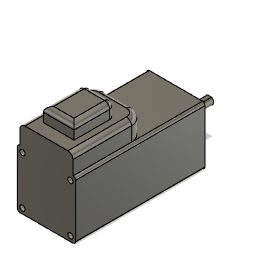
Mouting Plate BOB v17 (Autodesk Fusion 360 archive; units mm, degrees)
design "NEMA 23 Integrated Easy Servo Motor 130w"
Autodesk Fusion 360 part; units mm, degrees
sketch "Sketch1" plane through (0, 0, 0) normal (0, 0, 1) x (1, 0, 0)
  line L0 (0, 0) -> (57.15, 0)
  line L1 (57.15, 0) -> (57.15, 57.15)
  line L2 (57.15, 57.15) -> (0, 57.15)
  line L3 (0, 57.15) -> (0, 0)
  circle A0 centre (52.125, 52.125) radius 2.6
  line L4 (28.575, 0) -> (28.575, 57.15) construction
  line L5 (0, 28.575) -> (57.15, 28.575) construction
  circle A1 centre (5.025, 52.125) radius 2.6
  circle A2 centre (5.025, 5.025) radius 2.6
  circle A3 centre (52.125, 5.025) radius 2.6
  circle A4 centre (28.575, 28.575) radius 19.05
  line L6 (2.575, 57.15) -> (54.575, 57.15)
  line L7 (54.575, 57.15) -> (54.575, 76)
  line L8 (54.575, 76) -> (2.575, 76)
  line L9 (2.575, 76) -> (2.575, 57.15)
  circle A5 centre (28.575, 28.575) radius 4
  line L10 (26.6385, 32.075) -> (30.5115, 32.075)
  line L11 (13.575, 76) -> (43.575, 76)
  line L12 (43.575, 76) -> (43.575, 89.67)
  line L13 (43.575, 89.67) -> (13.575, 89.67)
  line L14 (13.575, 89.67) -> (13.575, 76)
  point P0 (47.5479, 45.3005)
  dimension "d1" = 57.15
  dimension "d2" = 57.15
  dimension "d3" = 5.2
  dimension "d5" = 5.2
  dimension "d6" = 47.1
  dimension "d8" = 5.2
  dimension "d10" = 47.1
  dimension "d12" = 5.2
  dimension "d13" = 47.1
  dimension "d14" = 47.1
  dimension "d15" = 38.1
  dimension "d16" = 76
  dimension "d17" = 8
  dimension "d19" = 3.5
  dimension "d20" = 52
  dimension "d21" = 13.67
  dimension "d22" = 30
  constraint horizontal L0
  constraint vertical L1
  constraint horizontal L2
  constraint vertical L3
  constraint coincident L0.start L3.end
  constraint midpoint L0 L4.start
  constraint midpoint L2 L4.end
  constraint midpoint L3 L5.start
  constraint midpoint L1 L5.end
  constraint symmetric A0 L4 A1
  constraint symmetric L5 A1.centre A2.centre
  constraint midpoint L5 A4.centre
  constraint horizontal L6
  constraint vertical L7
  constraint horizontal L8
  constraint vertical L9
  constraint coincident L2 L6.start
  constraint concentric A4 A5
  constraint coincident A5 L10.start
  constraint coincident A5 L10.end
  constraint perpendicular L4 L10
  constraint symmetric L4 L7 L9
  constraint horizontal L11
  constraint vertical L12
  constraint horizontal L13
  constraint vertical L14
  constraint coincident L8 L11.start
  constraint symmetric L4 L12 L14
  measures "d1" distance of L0.start L0.end
  measures "d2" distance of L0.start L2.end
  measures "d3" diameter of A0
  measures "d5" diameter of A1
  measures "d6" distance of A0.centre A1.centre
  measures "d8" diameter of A2
  measures "d10" distance of A1.centre A2.centre
  measures "d12" diameter of A3
  measures "d13" horizontal distance of A2.centre A3.centre
  measures "d14" distance of A0.centre A3.centre
  measures "d15" diameter of A4
  measures "d16" distance of L0 L8
  measures "d17" diameter of A5
  measures "d19" distance of L5 L10
  measures "d20" distance of L7.end L8.end
  measures "d21" distance of L11.start L13.end
  measures "d22" distance of L12.end L13.end
extrude "Extrude1" add sketch "Sketch1" along normal blind 127 contours L0 L1 L2 L3 L6 | A4 | A5 L10 | A5 L10
fillet "Fillet1" radius 2.5 4 edges at (57.15, 57.15, 63.5) (57.15, 0, 63.5) (0, 0, 63.5) (0, 57.15, 63.5)
extrude "Extrude2" add sketch "Sketch1" against normal blind 70 from surface at 127 contours L2 L6 L7 L8 L9 L11
fillet "Fillet2" radius 12.5 2 edges at (54.575, 66.575, 57) (2.575, 66.575, 57)
fillet "Fillet2" radius 5 3 edges at (54.575, 76, 92) (28.575, 76, 57) (2.575, 76, 92)
extrude "Extrude3" add sketch "Sketch1" along normal blind 40 from surface at 75 contours L8 L11 L12 L13 L14
fillet "Fillet3" radius 5 6 edges at (43.575, 89.67, 95) (43.575, 82.835, 75) (13.575, 82.835, 75) (28.575, 89.67, 75) (13.575, 89.67, 95) (28.575, 89.67, 115)
extrude "Extrude4" add sketch "Sketch1" against normal blind 2 contours A4 | A5 L10 | A5 L10
extrude "Extrude5" add sketch "Sketch1" against normal blind 33 contours A5 L10 picked at (29.5161, 29.5962)
extrude "Extrude6" add sketch "Sketch1" against normal blind 6 contours A5 L10 picked at (28.1041, 32.1557)
equation "d10 = d6"
equation "d12 = d3"
equation "d13 = d6"
equation "d14 = d6"
equation "d19 = 7.5 mm - ( d17 / 2 )"
equation "d44 = ( -1 * ( 33 - 27 ) ) * 1 mm"

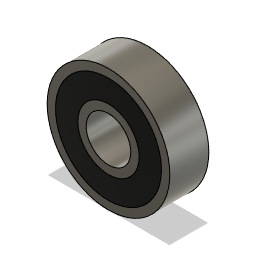
design "608 Bearings"
Autodesk Fusion 360 part; units mm, degrees
sketch "Sketch1" plane through (0, 0, 0) normal (0, 0, 1) x (1, 0, 0)
  circle A0 centre (0, 0) radius 11
  circle A1 centre (0, 0) radius 9.5
  circle A2 centre (0, 0) radius 4
  circle A3 centre (0, 0) radius 5.5
  dimension "d1" = 22
  dimension "d2" = -1.5
  dimension "d3" = 8
  dimension "d4" = 1.5
  constraint coincident A0.centre A1.centre
  measures "d1" diameter of A0
  measures "d3" diameter of A2
extrude "Extrude1" add sketch "Sketch1" along normal blind 7 makes body 1 at (5.4727, -0.5476, 4.6667) makes body 2 at (10.9453, -1.0952, 4.6667)
extrude "Extrude2" add sketch "Sketch1" along normal blind 7 separate body contours A1 makes body 3

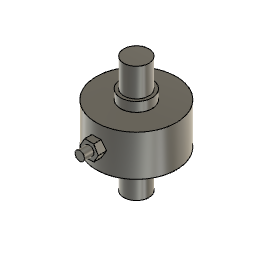
design "Load Cell Mini (200 kg)"
Autodesk Fusion 360 part; units mm, degrees
sketch "Boceto1" plane through (0, 0, 0) normal (0, 0, 1) x (1, 0, 0)
  circle A0 centre (0, 0) radius 12.7
  dimension "d1" = 25.4
  constraint coincident A0.centre origin
  measures "d1" diameter of A0
extrude "Extruir1" add sketch "Boceto1" along normal blind 13
sketch "Boceto2" plane through (0, 0, 13) normal (0, 0, 1) x (-1, 0, 0)
  circle A0 centre (0, 0) radius 12.7
  circle A1 centre (0, 0) radius 5
  dimension "d4" = 10
  constraint coincident A0.centre A1.centre
  measures "d4" diameter of A1
extrude "Extruir2" add sketch "Boceto2" along normal blind 3 contours A1
sketch "Boceto3" plane through (0, 0, 16) normal (0, 0, 1) x (-1, 0, 0)
  circle A0 centre (0, 0) radius 5
  circle A1 centre (0, 0) radius 4
  dimension "d7" = 8
  constraint coincident A0.centre A1.centre
  measures "d7" diameter of A1
extrude "Extruir3" add sketch "Boceto3" along normal blind 9 contours A1
sketch "Boceto4" plane through (0, 0, 0) normal (0, 0, -1) x (1, 0, 0)
  circle A0 centre (0, 0) radius 12.7
  circle A1 centre (0, 0) radius 4
  dimension "d10" = 8
  constraint coincident A0.centre A1.centre
  measures "d10" diameter of A1
extrude "Extruir4" add sketch "Boceto4" along normal blind 12 contours A1
sketch "Boceto5" plane through (0, 0, 0) normal (0, 1, 0) x (1, 0, 0)
  line L0 (-1.4434, -4) -> (-2.8868, -6.5)
  line L1 (-2.8868, -6.5) -> (-1.4434, -9)
  line L2 (-1.4434, -9) -> (1.4434, -9)
  line L3 (1.4434, -9) -> (2.8868, -6.5)
  line L4 (2.8868, -6.5) -> (1.4434, -4)
  line L5 (1.4434, -4) -> (-1.4434, -4)
  line L6 (-12.7, 0) -> (12.7, 0)
  point P0 (0, -6.5)
  dimension "d15" = 6.5
  dimension "d16" = 5
  measures "d15" distance of P0 L6
  measures "d16" distance of L2 L5
extrude "Extruir5" add sketch "Boceto5" against normal blind 15
sketch "Boceto6" plane through (0, -15, 0) normal (0, -1, 0) x (1, 0, 0)
  line L0 (-1.4434, 4) -> (1.4434, 4)
  line L1 (1.4434, 4) -> (2.8868, 6.5)
  line L2 (2.8868, 6.5) -> (1.4434, 9)
  line L3 (1.4434, 9) -> (-1.4434, 9)
  line L4 (-1.4434, 9) -> (-2.8868, 6.5)
  line L5 (-2.8868, 6.5) -> (-1.4434, 4)
  circle A0 centre (0, 6.5) radius 1.5
  dimension "d17" = 3
  measures "d17" diameter of A0
extrude "Extruir6" add sketch "Boceto6" along normal blind 3 contours A0

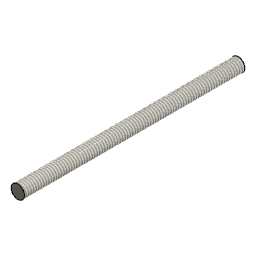
design "8mm T8 Lead Screw (130mm) v1"
Autodesk Fusion 360 part; units mm, degrees
sketch "Sketch1" plane through (0, 0, 0) normal (0, 0, 1) x (1, 0, 0)
  circle A0 centre (0, 0) radius 4
  dimension "d1" = 8
  constraint coincident A0.centre origin
  measures "d1" diameter of A0
extrude "Extrude1" add sketch "Sketch1" along normal blind 130
thread "Thread1" "ISO Metric Trapezoidal Threads 8.0 TR8x1.5 7e" major diameter 7.925 minor diameter 6.0605 pitch 1.5 angle 30 resizes the face on face at (3.9801, -0.3983, 43.3333)

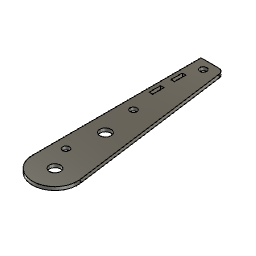
design "Pedal Inox"
Autodesk Fusion 360 part; units mm, degrees
sketch "Boceto1" plane through (0, 0, 0) normal (0, 0, 1) x (1, 0, 0)
  circle A0 centre (40.124, 0.0001) radius 5
  circle A1 centre (30, 20) radius 3
  line L0 (40.124, 0.0001) -> (40, -27.0971) construction
  line L1 (20.124, 0) -> (20.033, 149.9909)
  circle A2 centre (30, 80) radius 3
  line L2 (0, 0) -> (126.2621, 0) construction
  arc A3 (20.124, 0) -> (59.9438, 2.6787) centre (40.124, 0.0001) ccw
  line L3 (30, 149.997) -> (30, -50.821) construction
  circle A4 centre (35, 50) radius 5
  arc A5 (40.8406, 31.8952) -> (40.2572, 30.7033) centre (45, 29.1203) ccw
  line L4 (40.6186, 145.6701) -> (59.9438, 2.6787)
  line L5 (20.033, 149.9909) -> (35.6606, 150.0004)
  line L6 (23.4451, 129.993) -> (26.5451, 129.993)
  line L7 (26.5451, 129.993) -> (26.5451, 119.893)
  line L8 (26.5451, 119.893) -> (23.4451, 119.893)
  line L9 (23.4451, 119.893) -> (23.4451, 129.993)
  line L10 (26.5451, 100.493) -> (23.4451, 100.493)
  line L11 (26.5451, 110.593) -> (26.5451, 100.493)
  line L12 (23.4451, 100.493) -> (23.4451, 110.593)
  line L13 (23.4451, 110.593) -> (26.5451, 110.593)
  circle A6 centre (29.9988, 141.997) radius 3
  arc A7 (40.6186, 145.6701) -> (35.6606, 150.0004) centre (35.6637, 145.0004) ccw
  point P0 (20.033, 149.9909)
  point P1 (40.033, 150.0031)
  point P2 (40.033, 150.0031)
  dimension "d7" = 6
  dimension "d20" = 60
  dimension "d22" = 20
  dimension "d23" = 10
  dimension "d28" = 50
  dimension "d29" = 5
  dimension "d33" = 20
  dimension "d35" = 20
  dimension "d36" = 20
  dimension "d37" = 3.1
  dimension "d38" = 3.4
  dimension "d39" = 10.1
  dimension "d42" = 0
  dimension "d43" = -19.4
  dimension "d44" = 8
  dimension "d45" = 5
  constraint coincident P0 L1.end
  constraint equal A1 A2
  constraint coincident L2.start origin
  constraint horizontal L2
  constraint coincident A0.centre L0.start
  constraint concentric A0 A3
  constraint perpendicular L2 L3
  constraint equal A0 A4
  constraint tangent A3 L4
  constraint perpendicular L1 L5
  constraint horizontal L6
  constraint vertical L7
  constraint horizontal L8
  constraint vertical L9
  constraint coincident P2 L5
  constraint coincident L4 P2
  constraint tangent L5 A7
  constraint tangent L4 A7
  measures "d7" diameter of A1
  measures "d20" distance of A1.centre A2.centre
  measures "d22" radius of A3
  measures "d23" diameter of A0
  measures "d28" distance of L2 A4.centre
  measures "d29" distance of L3 A4.centre
  measures "d33" distance of P0 P2
  measures "d35" distance of P0 P2
  measures "d36" distance of L5 L6.start
  measures "d37" distance of L6.start L6.end
  measures "d38" distance of L1 L6.start
  measures "d39" distance of L6.start L8.end
  measures "d44" distance of L5 A6.centre
  measures "d45" radius of A7
extrude "Extruir1" add sketch "Boceto1" along normal blind 3

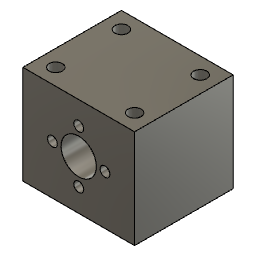
design "Lead Screw Nut Mount"
Autodesk Fusion 360 part; units mm, degrees
sketch "Sketch1" plane through (0, 0, 0) normal (0, 0, 1) x (1, 0, 0)
  circle A0 centre (0, 4) radius 5.375
  line L0 (-17, -11) -> (17, -11)
  line L1 (17, -11) -> (17, 19)
  line L2 (17, 19) -> (-17, 19)
  line L3 (-17, 19) -> (-17, -11)
  circle A1 centre (0, 12) radius 1.5
  circle A2 centre (-8, 4) radius 1.5
  circle A3 centre (0, -4) radius 1.5
  circle A4 centre (8, 4) radius 1.5
  dimension "d5" = 10.75
  dimension "d9" = 3
  dimension "d27" = 34
  dimension "d37" = 30
  constraint horizontal L0
  constraint vertical L1
  constraint horizontal L2
  constraint vertical L3
  measures "d5" diameter of A0
  measures "d9" diameter of A1
  measures "d27" distance of L1 L3
  measures "d37" distance of L0.end L1.end
extrude "Extrude1" add sketch "Sketch1" along normal blind 30
sketch "Sketch2" plane through (17, 0, 0) normal (1, 0, 0) x (0, 0, -1)
  line L0 (0, -11) -> (0, 19)
  line L1 (0, 19) -> (-30, 19)
  line L2 (-30, 19) -> (-30, -11)
  line L3 (-30, -11) -> (0, -11)
  circle A0 centre (-15, 44) radius 5
  line L4 (-15, 19) -> (-15, 44) construction
  circle A1 centre (-15, 44) radius 12.5
  line L5 (-30, 19) -> (-27.4409, 45.2145)
  line L6 (0, 19) -> (-2.5591, 45.2145)
  dimension "d20" = 10
  dimension "d35" = 25
  dimension "d36" = 25
  constraint midpoint L1 L4.start
  constraint perpendicular L1 L4
  constraint coincident A0.centre L4.end
  constraint concentric A0 A1
  constraint coincident L1.end L2.start
  constraint coincident A1 L5.end
  constraint tangent A1 L5
  constraint coincident L0.end L1.start
  constraint coincident A1 L6.end
  constraint tangent A1 L6
  measures "d20" diameter of A0
  measures "d35" distance of L4.start A0.centre
  measures "d36" diameter of A1
sketch "Boceto4" plane through (0, 19, 0) normal (0, 1, 0) x (-1, 0, 0)
  line L0 (-17, 0) -> (17, 0)
  line L1 (17, 0) -> (17, 30)
  line L2 (17, 30) -> (-17, 30)
  line L3 (-17, 30) -> (-17, 0)
  line L4 (-12, 25) -> (12, 25) construction
  line L5 (12, 25) -> (12, 5) construction
  line L6 (12, 5) -> (-12, 5) construction
  line L7 (-12, 5) -> (-12, 25) construction
  circle A0 centre (-12, 25) radius 2
  circle A1 centre (12, 25) radius 2
  circle A2 centre (12, 5) radius 2
  circle A3 centre (-12, 5) radius 2
  dimension "d40" = 24
  dimension "d41" = 20
  dimension "d42" = 5
  dimension "d43" = 5
  dimension "d44" = 4
  constraint horizontal L4
  constraint vertical L5
  constraint horizontal L6
  constraint vertical L7
  constraint coincident L4.start L7.end
  constraint coincident L4.end L5.start
  constraint coincident L5.end L6.start
  constraint coincident L6.end L7.start
  constraint equal A0 A3
  constraint equal A1 A3
  constraint equal A2 A3
  measures "d40" distance of L4.start L4.end
  measures "d41" distance of L4.end L5.end
  measures "d42" distance of L3 L7
  measures "d43" distance of L0 L6
  measures "d44" diameter of A3
extrude "Extruir4" cut sketch "Boceto4" against normal blind 4 contours A0 | A1 | A2 | A3
equation "Screw_Nut_Dia = 10 mm"
equation "Screw_Nut_bolt_Dia = 3 mm"
equation "Screw_Nut_Bolt_Pattern = 16 mm"
equation "d5 = Screw_Nut_Dia + 0.75 mm"
equation "d9 = Screw_Nut_bolt_Dia"
equation "d13 = Screw_Nut_bolt_Dia"
